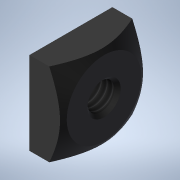
# Autodesk Inventor part: 25.50.0540
Saved by Autodesk Inventor 2021 (Build 250183000, 183)
## iProperties
Created: 2025-03-26
Part Number: 25.50.0540
Material: Generic
Catalog Web Link: www.cadenas.de
Description: Square Nut  M4-Series 25 with profile-grooves 6 mm
Vendor: MASCHINENBAUKITZ
Document SubType Name: Modeling
Designer: psAdmin
Manufacturer: MASCHINENBAUKITZ
Mass: 0.347892 g
Surface Area: 3.55633 cm^2
Volume: 0.347892 cm^3
Density: 1 g/cm^3
Appearance: PSOLRGB-191-191-191
Category: PARTsolutions
Company: MASCHINENBAUKITZ
Title: 25.50.0540
Author: Cadenas PARTsolutions
Comments: Series 25 with profile-grooves 6 mm
PSOL_IDENT_0: {$CADENAS_DATA/23d-libs/maschinenbau_kitz/1_profiltechnik/mk_verbinde/laschen/serie_25/25_50_0540.pr
PSOL_IDENT_1: j},168 {VTYP=3D},{NB=25.50.0540},{LINA=25.50.0540},{NN=Square Nut  M4},{DATE=02.05.2024 06:49:35},{G
PSOL_IDENT_2: EOMDATE=14.07.2023 10:11:46},{VERSION=},{LINEID=10},{WBVAR=},{WBNUMERIC=}  {NB=25.50.0540},{LINA=25.
PSOL_IDENT_3: 50.0540},{KT=DUMMY},{ARTIKELNR=25.50.0540},{BZ1=Mutter M4},{MTR=Stahl},{OBRFL=Verzinkt},{ABM=10 x 4
PSOL_IDENT_4: x 10 mm},{FRB=met. silber}
NB: 25.50.0540
NN: Square Nut  M4
NT: Series 25 with profile-grooves 6 mm
NBSYN: $ARTIKELNR.
LINA: 25.50.0540
CATALOG: Maschinenbau Kitz
ARTIKELNR: 25.50.0540
BZ1: Square Nut  M4
MTR: Steel
OBRFL: Zn
ABM: 10 x 4 x 10 mm
FRB: met. silver
SUPPLIER: MASCHINENBAUKITZ
ARTICLENO: 25.50.0540
BOMINFO: 25.50.0540
CREATOR: CADENAS GmbH
Autodesk Inventor part; units mm, degrees
ref_plane "YZ Plane" through (0, 0, 0) normal (1, 0, 0) x (0, 1, 0)
ref_plane "XZ Plane" through (0, 0, 0) normal (0, 1, 0) x (-1, 0, 0)
ref_plane "XY Plane" through (0, 0, 0) normal (0, 0, 1) x (1, 0, 0)
sketch "Skizze_1" plane through (0, 0, 0) normal (0, 0, 1) x (1, 0, 0)
  line L0 (4, 0) -> (0, 0)
  line L1 (0, 0) -> (0, 7.0725)
  line L2 (0, 7.0725) -> (2.3925, 7.0725)
  line L3 (2.3925, 7.0725) -> (4, 4.5)
  line L4 (4, 4.5) -> (4, 0)
  line L5 (4, 0) -> (0, 0)
  constraints: 12 end point
revolve "Revolution1" add sketch "Skizze_1" angle 360 about axis through (4, 0, 0) along (1, 0, 0)
sketch "Skizze_2" plane through (0, 0, 0) normal (0, 0, 1) x (1, 0, 0)
  line L0 (4, 0) -> (0, 0)
  line L1 (0, 0) -> (0, 2)
  line L2 (0, 2) -> (0.379, 1.621)
  line L3 (0.379, 1.621) -> (3.621, 1.621)
  line L4 (3.621, 1.621) -> (4, 2)
  line L5 (4, 2) -> (4, 0)
  line L6 (4, 0) -> (0, 0)
  constraints: 14 end point
revolve "Revolution2" cut sketch "Skizze_2" angle 360 about axis through (4, 0, 0) along (1, 0, 0)
thread "Thread1" size "M4x0.7" class "6H" standard "ISO Metric profile" full length
sketch "Skizze_3" plane through (0, 0, 0) normal (1, 0, 0) x (0, 1, 0)
  line L0 (10, 10) -> (-10, 10)
  line L1 (-10, 10) -> (-10, -10)
  line L2 (-10, -10) -> (10, -10)
  line L3 (10, -10) -> (10, 10)
  line L4 (5, 5) -> (-5, 5)
  line L5 (-5, 5) -> (-5, -5)
  line L6 (-5, -5) -> (5, -5)
  line L7 (5, -5) -> (5, 5)
  constraints: 16 end point
extrude "Extrusion1" cut sketch "Skizze_3" along normal blind 4
body "Solid1"
